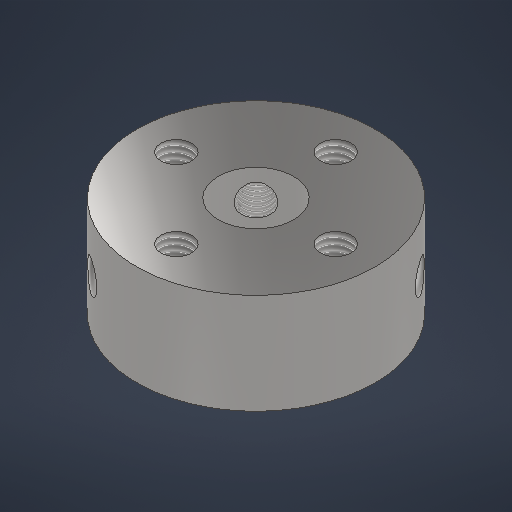
# Autodesk Inventor part: DiyHub
Saved by Autodesk Inventor 2027.1 (Build 311270010, 270A)
## iProperties
Created: 2026-04-20
Part Number: DiyHub
Material: Steel, Alloy
Document SubType Name: Modeling
Designer: szymo
Density: 7.73 g/cm^3
Appearance: Semi-Polished
Mass: 9.27765 g
Surface Area: 12.7709 cm^2
Volume: 1.20021 cm^3
Author: szymo
Autodesk Inventor part; units mm, degrees
ref_plane "XZ Plane" through (0, 0, 0) normal (0, 1, 0) x (-1, 0, 0)
sketch "Sketch1" plane through (0, 0, 0) normal (0, 1, 0) x (-1, 0, 0)
  circle A0 centre (0, 0) radius 15 construction
  circle A1 centre (0, 0) radius 9.5
  circle A2 centre (0, 0) radius 3
  circle A3 centre (0, 0) radius 6.35 construction
  circle A4 centre (6.35, 0) radius 3 construction
  line L0 (6.35, 0) -> (0, 0) construction
  circle A5 centre (6.35, 0) radius 2.5 construction
  circle A6 centre (0, 6.35) radius 2.5 construction
  circle A7 centre (0, 6.35) radius 3 construction
  circle A8 centre (-6.35, 0) radius 2.5 construction
  circle A9 centre (-6.35, 0) radius 3 construction
  circle A10 centre (0, -6.35) radius 2.5 construction
  circle A11 centre (0, -6.35) radius 3 construction
  point P0 (-1.9685, -4.5962)
  point P1 (-3.7402, -8.7328)
  point P2 (-4.5962, -1.9685)
  point P3 (-8.7328, -3.7402)
  point P4 (-4.5962, 1.9685)
  point P5 (-8.7328, 3.7402)
  point P6 (-1.9685, 4.5962)
  point P7 (-3.7402, 8.7328)
  point P8 (3.7402, 8.7328)
  point P9 (1.9685, 4.5962)
  point P10 (4.5962, 1.9685)
  point P11 (8.7328, 3.7402)
  point P12 (4.5962, -1.9685)
  point P13 (8.7328, -3.7402)
  point P14 (1.9685, -4.5962)
  point P15 (3.7402, -8.7328)
  dimension "d2" = 19
  dimension "d4" = 12.7
  dimension "d0" = 30
  dimension "d1" = 5.5
  dimension "d3" = 6
  dimension "d5" = 6
  dimension "d6" = 5
  dimension "d9" = 360
  constraints: 10 centre point, 8 coincident, 2 end point, 1 horizontal, 1 horizontal alignment, 29 other
  measures "d0" diameter of A0
  measures "d3" diameter of A2
  measures "d5" diameter of A4
  measures "d6" diameter of A5
extrude "Extrusion1" add sketch "Sketch1" against normal blind 1
extrude "Extrusion2" add sketch "Sketch1" against normal blind 8
hole "Hole1" at (-6.35, 0, 0) at (0, 0, -6.35) at (6.35, 0, 0) at (0, 0, 6.35) direction (0, -1, 0) diameter 2.459 depth 20 thread size "M3x0.5" class "6H" standard "ISO Metric profile"
ref_plane "Work Plane4" through (0, 0, 0) normal (0.7071068, 0, 0.7071068) x (0, 1, 0)
sketch "Sketch8" plane through (0, 0, 0) normal (0.7071068, 0, 0.7071068) x (0, 1, 0)
  line L0 (-8, -3) -> (-8, 3) construction
  line L1 (0, 3) -> (0, -3) construction
  line L2 (-8, -3) -> (0, -3) construction
  line L3 (-8, 3) -> (0, 3) construction
  line L4 (0, 0) -> (-8, 0) construction
  circle A0 centre (-2.25, 0) radius 1.25
  circle A1 centre (-5.75, 0) radius 1.25
  dimension "d92" = 2.5
  dimension "d93" = 2.5
  dimension "d94" = 1
  dimension "d95" = 1
  dimension "d96" = 1
  constraints: 2 centre point, 2 coincident, 2 end point, 2 point on line, 1 midpoint
  measures "d92" diameter of A0
  measures "d93" diameter of A1
  measures "d94" distance edge to line of A0 L1
  measures "d96" distance edge to line of A1 L0
hole "Hole9" at (0, -2.25, 0) at (0, -5.75, 0) direction (-0.7071068, 0, -0.7071068) diameter 2.459 depth 20 thread size "M3x0.5" class "6H" standard "ISO Metric profile"
sketch "Sketch9" plane through (0, 0, 0) normal (0, 1, 0) x (1, 0, 0)
  circle A0 centre (0, -6.35) radius 1.2295 projected
  circle A1 centre (6.35, 0) radius 1.2295 projected
  circle A2 centre (0, 6.35) radius 1.2295 projected
  circle A3 centre (-6.35, 0) radius 1.2295 projected
  circle A4 centre (0, 0) radius 9.5 projected
  circle A5 centre (0, 0) radius 3 projected
  line L0 (0, 0) -> (7.9468, 5.2056) construction
  line L1 (0, 0) -> (-5.2056, -7.9468) construction
  circle A6 centre (0, 0) radius 3 projected
  line L2 (2.9663, 0.4487) -> (8.5627, 4.1147)
  line L3 (1.5964, 2.54) -> (7.1928, 6.2059)
  line L4 (-2.54, -1.5964) -> (-6.2059, -7.1928)
  line L5 (-4.1147, -8.5627) -> (-0.4487, -2.9663)
  line L6 (1.5964, 2.54) -> (2.9663, 0.4487)
  line L7 (-0.4487, -2.9663) -> (-2.54, -1.5964)
  dimension "d97" = 1.25
  dimension "d98" = 1.25
  dimension "d99" = 1.25
  dimension "d100" = 1.25
  dimension "d101" = 1
  dimension "d102" = 1
  constraints: 16 end point, 10 point on circle, 4 parallel
  measures "d97" distance between parallel lines of L1 L5
  measures "d98" distance between parallel lines of L1 L4
  measures "d99" distance between parallel lines of L0 L2
  measures "d100" distance between parallel lines of L3 L0
  measures "d101" distance edge to line of A1 L2
  measures "d102" distance edge to line of A0 L5
ref_plane "Work Plane5" through (1.5964, 0, -2.54) normal (0.8365093, 0, -0.5479528) x (0.5479528, 0, 0.8365093)
ref_plane "Work Plane6" through (-0.4487, 0, 2.9663) normal (-0.5479528, 0, 0.8365093) x (-0.8365093, 0, -0.5479528)
sketch "Sketch10" plane through (1.5964, 0, -2.54) normal (0.8365093, 0, -0.5479528) x (0.5479528, 0, 0.8365093)
  line L0 (-1.75, 8) -> (4.25, 8) projected
  line L1 (4.25, 0) -> (-1.75, 0) projected
  line L2 (4.25, 0) -> (-1.75, 0) projected
  line L3 (4.25, 0) -> (-1.75, 8)
  line L4 (-1.75, 8) -> (4.25, 8) projected
  line L5 (4.25, 8) -> (-1.75, 0)
  point P0 (1.25, 0)
  point P1 (1.25, 4)
  constraints: 4 end point, 1 midpoint, 2 other
hole "Hole10" at (2.2813, -4, -1.4944) direction (0.8365093, 0, -0.5479528) diameter 2.459 depth 20 thread size "M3x0.5" class "6H" standard "ISO Metric profile"
sketch "Sketch11" plane through (-0.4487, 0, 2.9663) normal (-0.5479528, 0, 0.8365093) x (-0.8365093, 0, -0.5479528)
  line L0 (-1.75, 8) -> (4.25, 8) construction
  line L1 (4.25, 0) -> (-1.75, 0) construction
  line L2 (4.25, 0) -> (-1.75, 8) construction
  line L3 (4.25, 8) -> (-1.75, 0) construction
  point P0 (1.25, 0)
  point P1 (1.25, 4)
  constraints: 4 end point, 1 midpoint, 3 other
hole "Hole11" at (-1.4944, -4, 2.2813) direction (-0.5479528, 0, 0.8365093) diameter 2.459 depth 20 thread size "M3x0.5" class "6H" standard "ISO Metric profile"
equation "\"d93\" = d92"
equation "\"d94\" = d96"
equation "\"d95\" = d96"
equation "\"d98\" = d97"
equation "\"d99\" = d97"
equation "\"d100\" = d97"
equation "\"d102\" = d101"
body "Solid1"
